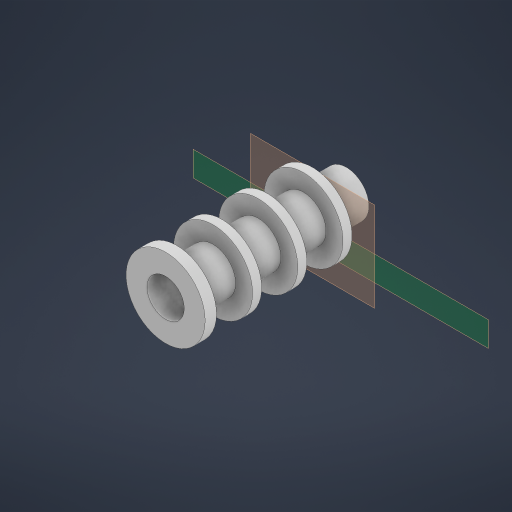
# Autodesk Inventor part: puleggia
Saved by Autodesk Inventor 2024.3 (Build 283343000, 343)
## iProperties
Created: 2025-08-20
Part Number: puleggia
Material: Generic
Document SubType Name: Modeling
Designer: giuseppe
Density: 1 g/cm^3
Appearance: Default
Author: giuseppe
## iProperties of the stored document puleggia_3DPrint.ipt
Created: 2025-08-21
Part Number: puleggia_3DPrint
Material: Generic
Document SubType Name: Modeling
Designer: giuseppe
Density: 1 g/cm^3
Appearance: Default
Author: giuseppe
Autodesk Inventor part; units mm, degrees
ref_plane "YZ Plane" through (0, 0, 0) normal (1, 0, 0) x (0, 1, 0)
ref_plane "XZ Plane" through (0, 0, 0) normal (0, 1, 0) x (-1, 0, 0)
ref_plane "XY Plane" through (0, 0, 0) normal (0, 0, 1) x (1, 0, 0)
sketch "Sketch1" plane through (0, 0, 0) normal (0, 0, 1) x (1, 0, 0)
  circle A0 centre (0, -2.5) radius 1.25 construction
  circle A1 centre (0, -2.5) radius 2
  point P0 (0, 0)
  dimension "d0" = 4
  constraints: 1 centre point, 1 concentric
  measures "d0" diameter of A1
extrude "Extrusion1" add sketch "Sketch1" along normal blind 15
ref_plane "Work Plane1" through (10.522, -7.5, 0.5) normal (0, 0, -1) x (1, 0, 0)
sketch "Sketch3" plane through (0, -2.5, 15) normal (0, 0, 1) x (1, 0, 0)
  circle A0 centre (0, 0) radius 3.5
  circle A1 centre (0, 0) radius 2 projected
  point P0 (0, 2.5)
  dimension "d7" = 1.5
  constraints: 1 centre point, 1 concentric
  measures "d7" radial gap between concentric circles of A0 A1
extrude "Extrusion3" add sketch "Sketch3" along normal blind 1 contours A0 | A1
sketch "Sketch4" plane through (0, -2.5, 16) normal (0, 0, 1) x (1, 0, 0)
  circle A0 centre (0, 0) radius 1.65
  circle A1 centre (0, 0) radius 3.5 projected
  point P0 (0, 2.5)
  dimension "d10" = 3.3
  constraints: 1 centre point, 1 concentric
  measures "d10" diameter of A0
extrude "Extrusion4" cut sketch "Sketch4" against normal through all contours A0
ref_plane "Work Plane2" through (0, -4, 3) normal (0, 0, 1) x (-1, 0, 0)
sketch "Sketch5" plane through (0, -4, 3) normal (0, 0, 1) x (-1, 0, 0)
  circle A0 centre (0, -1.5) radius 3.5 projected
  circle A1 centre (0, -1.5) radius 1.65 projected
  circle A2 centre (0, -1.5) radius 3.5 projected
  point P0 (0, -4)
extrude "Extrusion5" add sketch "Sketch5" along normal blind 0.8
pattern_linear "Rectangular Pattern1" count 3 spacing 4 along (0, 0, 1) of "Extrusion5"
body "Solid1"
